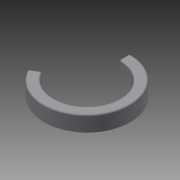
# Autodesk Inventor part: Top
Saved by Autodesk Inventor 2015 (Build 190159000, 159)
## iProperties
Created: 2016-03-23
Part Number: Top
Material: Generic
Document SubType Name: Modeling
Designer: david_000
Density: 1 g/cm^3
Appearance: Default
Author: david_000
Autodesk Inventor part; units mm, degrees
ref_plane "YZ Plane" through (0, 0, 0) normal (1, 0, 0) x (0, 1, 0)
ref_plane "XZ Plane" through (0, 0, 0) normal (0, 1, 0) x (-1, 0, 0)
ref_plane "XY Plane" through (0, 0, 0) normal (0, 0, 1) x (1, 0, 0)
sketch "Sketch1" plane through (0, 0, 0) normal (1, 0, 0) x (0, 1, 0)
  line L0 (0.2223, 0) -> (56.1023, 0)
  line L1 (56.1023, 0) -> (56.1023, -44.45)
  line L2 (56.1023, -44.45) -> (-7.3977, -44.45)
  line L3 (-7.3977, -44.45) -> (-7.3977, -42.8625)
  line L4 (-7.3977, -42.8625) -> (-10.5727, -42.8625)
  line L5 (-10.5727, -42.8625) -> (-10.5727, -41.275)
  line L6 (-10.5727, -41.275) -> (52.9273, -41.275)
  line L7 (52.9273, -41.275) -> (52.9273, -3.175)
  line L8 (52.9273, -3.175) -> (0.2223, -3.175)
  line L9 (0.2223, -3.175) -> (0.2223, 0)
  line L10 (68.5874, 139.7) -> (-16.5119, 139.7)
  point P0 (0, 0)
  dimension "d0" = 55.88
  dimension "d1" = 44.45
  dimension "d2" = 63.5
  dimension "d3" = 1.5875
  dimension "d4" = 90
  dimension "d5" = 3.175
  dimension "d6" = 1.5875
  dimension "d7" = 63.5
  dimension "d8" = 38.1
  dimension "d9" = 90
  dimension "d10" = 139.7
  constraints: 22 end point, 9 perpendicular, 2 horizontal
  measures "d0" distance of L0.start L0.end
  measures "d1" distance of L0.end L1.end
  measures "d2" distance of L1.end L2.end
  measures "d3" distance of L2.end L3.end
  measures "d4" angle of L2 L3
  measures "d5" distance of L3.end L4.end
  measures "d6" distance of L4.end L5.end
  measures "d7" distance of L5.end L6.end
  measures "d8" distance of L6.end L7.end
  measures "d9" angle of L7 L6
  measures "d10" distance between parallel lines of L0 L10
revolve "Revolution1" add sketch "Sketch1" angle 240 about axis through (0, 68.5874, 139.7) along (0, -1, 0)
fillet "Fillet1" radius 6.35 1 edges at (159.4786, 56.1023, 231.775)
fillet "Fillet2" radius 6.35 1 edges at (120.9837, 56.1023, 209.55)
body "Solid1"
